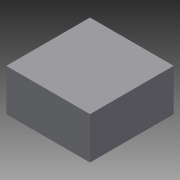
# Autodesk Inventor part: router
Saved by Autodesk Inventor 2015 (Build 190159000, 159)
## iProperties
Created: 2015-11-07
Part Number: router
Material: Generic
Document SubType Name: Modeling
Designer: Jufo
Density: 1 g/cm^3
Appearance: Default
Author: Jufo
Autodesk Inventor part; units mm, degrees
ref_plane "YZ Plane" through (0, 0, 0) normal (1, 0, 0) x (0, 1, 0)
ref_plane "XZ Plane" through (0, 0, 0) normal (0, 1, 0) x (-1, 0, 0)
ref_plane "XY Plane" through (0, 0, 0) normal (0, 0, 1) x (1, 0, 0)
sketch "Sketch1" plane through (0, 0, 0) normal (0, 1, 0) x (-1, 0, 0)
  line L0 (55.6862, 32.1373) -> (55.6862, -25.8627)
  line L1 (55.6862, -25.8627) -> (-2.3138, -25.8627)
  line L2 (-2.3138, -25.8627) -> (-2.3138, 32.1373)
  line L3 (-2.3138, 32.1373) -> (55.6862, 32.1373)
  point P0 (0, 0)
  dimension "d0" = 58
  dimension "d1" = 58
  constraints: 8 end point, 3 perpendicular, 1 vertical
  measures "d0" distance of L0.start L0.end
  measures "d1" distance of L0.end L1.end
extrude "Extrusion1" add sketch "Sketch1" along normal blind 29
body "Solid1"
